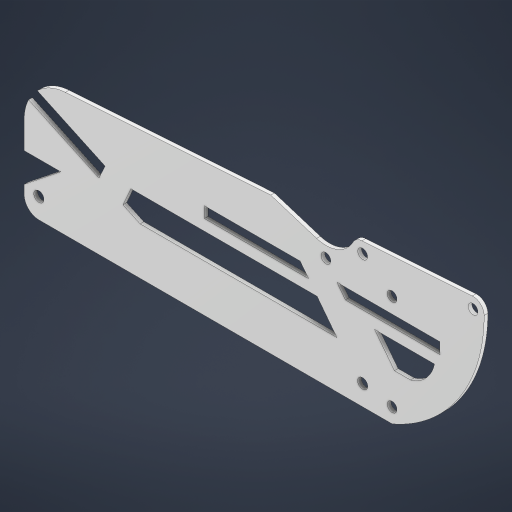
# Autodesk Inventor part: sled
Saved by Autodesk Inventor 2024 (Build 280153000, 153)
## iProperties
Created: 2023-11-03
Part Number: sled
Material: Acetal Resin, White
Document SubType Name: Sheet Metal
Designer: avere
Density: 1.425 g/cm^3
Appearance: Smooth - White
Flat Pattern Width: 6.50875 cm
Flat Pattern Length: 19.8438 cm
Flat Pattern Area: 129.158 cm^2
Sheet Metal Rule: Default_mm
Sheet Metal Width: 2.563 in
Sheet Metal Length: 7.813 in
Sheet Metal Area: 20.020 in^2
Author: avere
Autodesk Inventor part; units mm, degrees
ref_plane "YZ Plane" through (0, 0, 0) normal (1, 0, 0) x (0, 1, 0)
ref_plane "XZ Plane" through (0, 0, 0) normal (0, 1, 0) x (-1, 0, 0)
ref_plane "XY Plane" through (0, 0, 0) normal (0, 0, 1) x (1, 0, 0)
sketch "Sketch1" plane through (0, 0, 0) normal (0, 0, 1) x (1, 0, 0)
  circle A0 centre (0, 0) radius 2.0955
  arc A1 (0, -6.35) -> (2.9931, -5.6004) centre (0, 0) ccw
  arc A2 (-158.75, 0) -> (-152.4, -6.35) centre (-152.4, 0) ccw
  line L0 (-152.4, -6.35) -> (0, -6.35)
  line L1 (-158.75, 28.575) -> (-158.75, 22.225)
  circle A3 centre (-12.7, 2.3813) radius 2.1844
  circle A4 centre (-152.4, 2.3813) radius 2.1844
  circle A5 centre (0, 41.275) radius 2.0955
  circle A6 centre (34.925, 53.975) radius 2.0955
  arc A7 (39.6875, 53.9822) -> (34.6082, 58.727) centre (34.925, 53.975) ccw
  arc A8 (0, -6.35) -> (39.6875, 53.9822) centre (-25.8638, 53.8832) ccw
  circle A9 centre (-12.7, 50.8) radius 2.0955
  arc A10 (-13.0168, 55.552) -> (-16.9032, 53.0393) centre (-12.7, 50.8) ccw
  circle A11 centre (-28.5752, 41.2702) radius 2.0955
  arc A12 (-32.5685, 46.65) -> (-16.9032, 53.0393) centre (-28.5752, 59.2579) ccw
  line L2 (-32.5685, 46.65) -> (-52.3875, 52.9272)
  line L3 (34.6082, 58.727) -> (-13.0168, 55.552)
  line L4 (-52.3875, 52.9272) -> (-140.9672, 47.0219)
  line L5 (-153.0722, 41.582) -> (-123.825, 28.0141)
  line L6 (-123.825, 28.0141) -> (-126.4972, 22.2538)
  line L7 (-80.9625, 34.6421) -> (-80.9625, 29.8796)
  line L8 (20.6375, 29.8796) -> (20.6375, 34.6421)
  line L9 (-116.1342, 17.4463) -> (-112.7125, 25.1339)
  line L10 (-112.7125, 25.1339) -> (-32.3729, 25.1339)
  line L11 (-7.5532, 25.1339) -> (18.2795, 25.1339)
  line L12 (7.9375, 14.0071) -> (1.0071, 14.0071)
  line L13 (-23.8127, 14.0071) -> (-108.7205, 14.0071)
  line L14 (-80.9625, 29.8796) -> (-36.0239, 29.8796)
  line L15 (-20.1488, 29.8796) -> (20.6375, 29.8796)
  line L16 (-23.8127, 14.0071) -> (-32.3729, 25.1339)
  line L17 (-36.0239, 29.8796) -> (-39.6879, 34.6421)
  line L18 (20.6375, 34.6421) -> (-23.8127, 34.6421)
  line L19 (-39.6879, 34.6421) -> (-80.9625, 34.6421)
  line L20 (1.0071, 14.0071) -> (-7.5532, 25.1339)
  line L21 (-20.1488, 29.8796) -> (-23.8127, 34.6421)
  arc A13 (-140.9672, 47.0219) -> (-153.0722, 41.582) centre (-139.7, 28.0141) ccw
  arc A14 (-156.8393, 36.3296) -> (-158.75, 28.0141) centre (-139.7, 28.0141) ccw
  line L22 (-108.7205, 14.0071) -> (-116.1342, 17.4463)
  line L23 (-126.4972, 22.2538) -> (-156.8393, 36.3296)
  line L24 (-158.75, 3.7399) -> (-147.5087, 12.7329)
  line L25 (-158.75, 3.7399) -> (-142.9797, 16.3561)
  line L26 (-142.9797, 16.3561) -> (-158.75, 16.3561)
  line L27 (-158.75, 28.0141) -> (-158.75, 16.3561)
  line L28 (-158.75, 3.7399) -> (-158.75, 0)
  arc A15 (7.9375, 14.0071) -> (18.2795, 25.1339) centre (3.9598, 28.0739) ccw
  dimension "d36" = 4.191
  dimension "d52" = 4.3688
  dimension "d53" = 4.3688
  dimension "d54" = 4.191
  dimension "d57" = 4.191
  dimension "d59" = 4.191
  dimension "d63" = 4.191
  dimension "d66" = 4.7625
  dimension "d70" = 20.1958
  constraints: 58 end point, 18 point on circle, 16 centre point, 14 tangent, 11 perpendicular, 8 parallel, 3 coincident, 2 horizontal, 2 point on line, 4 other
  measures "d36" diameter of A0
  measures "d52" diameter of A3
  measures "d53" diameter of A4
  measures "d54" diameter of A5
  measures "d57" diameter of A6
  measures "d59" diameter of A9
  measures "d63" diameter of A11
  measures "d66" distance of L7.start L7.end
  measures "d70" distance of L24.start L25.end
extrude "Extrusion1" add sketch "Sketch1" along normal blind 1.5875
equation "\"BendRadius\" = Thickness"
equation "\"BendReliefWidth\" = Thickness"
equation "\"BendReliefDepth\" = 0.5 * Thickness"
equation "\"CornerReliefSize\" = 4 * Thickness"
equation "\"MinimumRemnant\" = 2 * Thickness"
equation "\"TransitionRadius\" = BendRadius"
equation "\"JacobiRadiusSize\" = BendRadius"
equation "\"GapSize\" = Thickness"
equation "\"Thickness\" = 1.5875"
body "Solid1"
